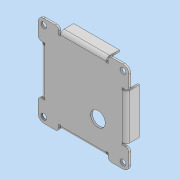
# Autodesk Inventor part: WaageBlechOberseite
Saved by Autodesk Inventor 2022 (Build 260153000, 153)
## iProperties
Created: 2021-12-03
Part Number: WaageBlechOberseite
Material: Generic
Document SubType Name: Sheet Metal
Designer: domin
Density: 1 g/cm^3
Sheet Metal Rule: Default_mm
Appearance: Default
Author: domin
Autodesk Inventor part; units mm, degrees
note: some values were not read from the file. Chosen so that the rebuilt part matches the saved one: relief shape of "Plate2".
ref_plane "YZ Plane" through (0, 0, 0) normal (1, 0, 0) x (0, 1, 0)
ref_plane "XZ Plane" through (0, 0, 0) normal (0, 1, 0) x (-1, 0, 0)
ref_plane "XY Plane" through (0, 0, 0) normal (0, 0, 1) x (1, 0, 0)
sketch "Sketch2" plane through (0, 0, 0) normal (0, 0, 1) x (1, 0, 0)
  line L0 (-78.5, 42.5) -> (-74, 42.5)
  line L1 (-74, 42.5) -> (-74, -42.5)
  line L2 (-74, -42.5) -> (-78.5, -42.5)
  line L3 (-78.5, -78.5) -> (-78.5, -42.5)
  line L4 (-78.5, 42.5) -> (-78.5, 78.5)
  line L5 (42.5, 78.5) -> (42.5, 74)
  line L6 (42.5, 74) -> (-42.5, 74)
  line L7 (-42.5, 74) -> (-42.5, 78.5)
  line L8 (78.5, 42.5) -> (74, 42.5)
  line L9 (74, 42.5) -> (74, -42.5)
  line L10 (74, -42.5) -> (78.5, -42.5)
  line L11 (42.5, -78.5) -> (42.5, -74)
  line L12 (42.5, -74) -> (-42.5, -74)
  line L13 (-42.5, -74) -> (-42.5, -78.5)
  line L14 (78.5, 78.5) -> (78.5, 42.5)
  line L15 (78.5, -42.5) -> (78.5, -78.5)
  line L16 (-78.5, 78.5) -> (-42.5, 78.5)
  line L17 (42.5, 78.5) -> (78.5, 78.5)
  line L18 (78.5, -78.5) -> (42.5, -78.5)
  line L19 (-42.5, -78.5) -> (-78.5, -78.5)
  point P0 (0, 0)
  dimension "d5" = 157
  dimension "d6" = 157
  dimension "d7" = 36
  dimension "d8" = 78.5
  dimension "d9" = 148
  dimension "d10" = 74
  dimension "d11" = 148
  dimension "d12" = 74
  dimension "d13" = 78.5
  dimension "d14" = 36
  measures "d5" distance between parallel lines of L14 L4
  measures "d6" distance between parallel lines of L19 L16
  measures "d7" distance between parallel lines of L0 L16
  measures "d8" distance from line of point (0, 0) L16
  measures "d9" distance between parallel lines of L9 L1
  measures "d10" distance from line of point (0, 0) L1
  measures "d11" distance between parallel lines of L12 L6
  measures "d12" distance from line of point (0, 0) L6
  measures "d13" distance from line of L4 point (0, 0)
  measures "d14" distance between parallel lines of L7 L4
extrude "Plate1" add sketch "Sketch2" along normal blind 3
sketch "Sketch3" plane through (-71, 42.5, 3) normal (-1, 0, 0) x (0, -1, 0)
  line L0 (82, 0) -> (3, 0)
  line L1 (3, 0) -> (3, -22.5)
  line L2 (3, -22.5) -> (82, -22.5)
  line L3 (82, -22.5) -> (82, 0)
  constraints: 8 end point
edge flange "Flange1" height 22.5 angle 90 thickness 3 bend radius 3 thickness toward (-1, 0, 0) relief straight relief width 3 relief depth 1.5 corner gap 3 corner form 0 edges at (-74, 0, 0) (0, -74, 0) (74, 0, 0) (0, 74, 0) wall of the first edge with corners at (-71, -39.5, 3) (-71, 39.5, 3) (-71, 39.5, -19.5) (-71, -39.5, -19.5)
bend "Bend1"
corner "Corner1"
fillet "Corner Round1" radius 6 8 edges at (78.5, -42.5, 1.5) (42.5, -78.5, 1.5) (-42.5, -78.5, 1.5) (-78.5, -42.5, 1.5) (-78.5, 42.5, 1.5) (-42.5, 78.5, 1.5) (42.5, 78.5, 1.5) (78.5, 42.5, 1.5)
fillet "Corner Round2" radius 10 4 edges at (78.5, -78.5, 1.5) (78.5, 78.5, 1.5) (-78.5, 78.5, 1.5) (-78.5, -78.5, 1.5)
sketch "Sketch4" plane through (0, 0, 3) normal (0, 0, 1) x (1, 0, 0)
  line L0 (68.475, -68.475) -> (-68.475, -68.475)
  line L1 (-68.475, -68.475) -> (-68.475, 68.475)
  line L2 (-68.475, 68.475) -> (68.475, 68.475)
  line L3 (68.475, 68.475) -> (68.475, -68.475)
  circle A0 centre (68.475, -68.475) radius 4.875
  point P0 (0, 0)
  dimension "d28" = 136.95
  dimension "d29" = 136.95
  dimension "d30" = 68.475
  dimension "d31" = 68.475
  dimension "d32" = 9.75
  constraints: 8 end point, 2 parallel, 1 centre point, 1 coincident, 1 horizontal, 1 perpendicular
  measures "d28" distance of L0.start L0.end
  measures "d29" distance between parallel lines of L2 L0
  measures "d30" distance from line of point (0, 0) L3
  measures "d31" distance from line of point (0, 0) L0
  measures "d32" diameter of A0
hole "Hole1" at (68.475, -68.475, 3) at (-68.475, -68.475, 3) at (-68.475, 68.475, 3) at (68.475, 68.475, 3) direction (0, 0, -1) diameter 9.75 end through all
sketch "Sketch5" plane through (0, 0, 3) normal (0, 0, 1) x (1, 0, 0)
  circle A0 centre (25, -25) radius 12.5
  point P0 (0, 0)
  dimension "d40" = 25
  dimension "d41" = 25
  dimension "d42" = 25
  constraints: 1 centre point
  measures "d40" diameter of A0
  measures "d41" horizontal distance of point (0, 0) A0.centre
  measures "d42" horizontal distance of point (0, 0) A0.centre
extrude "Cut1" cut sketch "Sketch5" against normal blind 3
equation "\"d29\" = d28"
equation "\"d30\" = 0.5 * d28"
equation "\"d31\" = 0.5 * d29"
equation "\"d33\" = d32"
equation "\"d38\" = Thickness"
equation "\"d43\" = Thickness"
equation "\"d15\" = Thickness"
equation "\"d16\" = BendReliefWidth"
equation "\"d17\" = BendReliefDepth"
equation "\"d18\" = MinimumRemnant"
equation "\"d19\" = TransitionRadius"
equation "\"d22\" = BendRadius"
equation "\"d23\" = CornerReliefSize"
equation "\"d24\" = GapSize"
equation "\"d25\" = JacobiRadiusSize"
equation "\"d10\" = 0.5 * d9"
equation "\"d12\" = 0.5 * d11"
equation "\"BendRadius\" = Thickness"
equation "\"BendReliefWidth\" = Thickness"
equation "\"BendReliefDepth\" = 0.5 * Thickness"
equation "\"CornerReliefSize\" = 4 * Thickness"
equation "\"MinimumRemnant\" = 2 * Thickness"
equation "\"TransitionRadius\" = BendRadius"
equation "\"JacobiRadiusSize\" = BendRadius"
equation "\"GapSize\" = Thickness"
equation "\"d2\" = 0.5 * d1"
equation "\"d3\" = 0.5 * d0"
equation "\"Thickness\" = 3"
equation "\"d1\" = 157"
equation "\"d0\" = 157"
body "Solid1"
